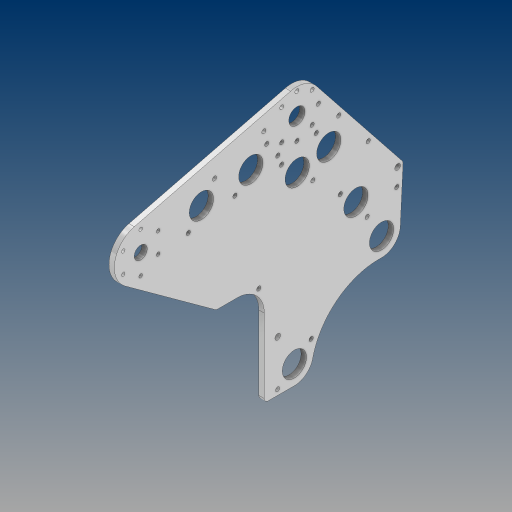
# Autodesk Inventor part: Intake Roller Plate
Saved by Autodesk Inventor 2024.3 (Build 283343000, 343)
## iProperties
Created: 2024-07-25
Part Number: Intake Roller Plate
Material: Aluminum 6061
Document SubType Name: Modeling
Designer: Kenji
Density: 2.7 g/cm^3
Appearance: Aluminum - Dark
Author: Kenji
Autodesk Inventor part; units mm, degrees
ref_plane "YZ Plane" through (0, 0, 0) normal (1, 0, 0) x (0, 1, 0)
ref_plane "XZ Plane" through (0, 0, 0) normal (0, 1, 0) x (-1, 0, 0)
ref_plane "XY Plane" through (0, 0, 0) normal (0, 0, 1) x (1, 0, 0)
sketch "Sketch1" plane through (0, 0, 0) normal (1, 0, 0) x (0, 1, 0)
  line L0 (127, 0) -> (127, -31.75) construction
  line L1 (95.25, -63.5) -> (31.75, -63.5) construction
  line L2 (0, -31.75) -> (0, 0) construction
  arc A0 (95.25, -63.5) -> (127, -31.75) centre (95.25, -31.75) ccw construction
  arc A1 (0, -31.75) -> (31.75, -63.5) centre (31.75, -31.75) ccw construction
  line L3 (0, 0) -> (0, 19.05) construction
  line L4 (0, 19.05) -> (-12.7, 19.05) construction
  line L5 (82.55, 19.05) -> (82.55, 292.1) construction
  circle A2 centre (82.55, 292.1) radius 25.4 construction
  circle A3 centre (82.55, 292.1) radius 31.75 construction
  circle A4 centre (231.775, 292.1) radius 25.4 construction
  circle A5 centre (231.775, 292.1) radius 31.75 construction
  line L6 (-12.7, 19.05) -> (82.55, 19.05) construction
  line L7 (127, 0) -> (0, 0) construction
  line L8 (-12.7, 19.05) -> (-12.7, -285.75) construction
  circle A6 centre (38.1, -172.5837) radius 50.8 construction
  circle A7 centre (104.9083, -202.0677) radius 25.4 construction
  circle A8 centre (104.9083, -202.0677) radius 14.2875
  circle A9 centre (154.8209, -171.8196) radius 25.4 construction
  circle A10 centre (154.8209, -171.8196) radius 14.2875
  circle A11 centre (250.0002, -47.5843) radius 22.225 construction
  circle A12 centre (250.0002, -47.5843) radius 25.4 construction
  circle A13 centre (250.0002, -47.5843) radius 14.2875
  line L9 (82.55, 19.05) -> (127, 19.05) construction
  line L10 (127, 19.05) -> (127, 0) construction
  circle A14 centre (154.8209, -171.8196) radius 22.225 construction
  circle A15 centre (104.9083, -202.0677) radius 22.225 construction
  circle A16 centre (25.4, -99.06) radius 25.4 construction
  circle A17 centre (25.4, -99.06) radius 23.8125 construction
  line L11 (25.4, -73.66) -> (25.4, -63.5) construction
  circle A18 centre (219.8086, -102.3786) radius 25.4 construction
  circle A19 centre (219.8086, -102.3786) radius 22.225 construction
  circle A20 centre (219.8086, -102.3786) radius 14.2875
  line L12 (0, -99.06) -> (-12.7, -99.06) construction
  circle A21 centre (63.172, -79.375) radius 6.477 construction
  circle A22 centre (25.4, -99.06) radius 14.2875
  circle A23 centre (63.172, -79.375) radius 3.2512
  circle A24 centre (95.1707, -129.6948) radius 50.8 construction
  circle A25 centre (147.0613, -96.0158) radius 50.8 construction
  circle A26 centre (105.4747, -117.9903) radius 50.8 construction
  circle A27 centre (166.1747, -221.0415) radius 3.2512
  circle A28 centre (242.3971, 10.8357) radius 14.2875
  circle A29 centre (242.3971, 10.8357) radius 22.225 construction
  line L13 (219.8086, -102.3786) -> (154.8209, -171.8196) construction
  line L14 (154.8209, -171.8196) -> (104.9083, -202.0677) construction
  line L15 (82.55, 19.05) -> (31.75, 19.05) construction
  line L16 (31.75, 19.05) -> (31.75, 292.1) construction
  line L17 (31.75, 292.1) -> (82.55, 292.1) construction
  circle A30 centre (242.3971, 10.8357) radius 7.62 construction
  line L18 (-12.7, -285.75) -> (571.5, -285.75) construction
  line L19 (571.5, -285.75) -> (571.5, 292.1) construction
  line L20 (31.75, 292.1) -> (571.5, 292.1) construction
  line L21 (127, 19.05) -> (571.5, 19.05) construction
  circle A31 centre (230.3321, 82.55) radius 7.62
  circle A32 centre (230.3321, 82.55) radius 23.8125 construction
  circle A33 centre (254.1446, 82.55) radius 2.0828
  circle A34 centre (230.3321, 82.55) radius 27.94 construction
  circle A35 centre (230.3321, 82.55) radius 31.115 construction
  circle A36 centre (242.2384, 103.1722) radius 2.0828
  circle A37 centre (218.4259, 103.1722) radius 2.0828
  circle A38 centre (206.5196, 82.55) radius 2.0828
  circle A39 centre (218.4259, 61.9278) radius 2.0828
  circle A40 centre (242.2384, 61.9278) radius 2.0828
  line L22 (-12.7, -63.5) -> (368.3, -63.5) construction
  circle A41 centre (166.1747, -221.0415) radius 6.4262 construction
  line L23 (368.3, -63.5) -> (368.3, -285.75) construction
  circle A42 centre (63.172, -79.375) radius 6.35 construction
  circle A43 centre (242.3971, 10.8357) radius 25.4 construction
  line L24 (242.3971, 10.8357) -> (250.0002, -47.5843) construction
  line L25 (82.55, 19.05) -> (141.3002, 19.05) construction
  line L26 (141.3002, 19.05) -> (141.3002, 209.55) construction
  line L27 (141.3002, 209.55) -> (82.55, 209.55) construction
  line L28 (82.55, 209.55) -> (82.55, 19.05) construction
  circle A44 centre (133.35, 12.7) radius 6.35 construction
  circle A45 centre (177.4795, -39.017) radius 50.8 construction
  circle A46 centre (177.8, -23.221) radius 50.8 construction
  circle A47 centre (25.4, -99.06) radius 22.225 construction
  line L29 (3.175, -99.06) -> (3.175, -68.2752)
  circle A48 centre (133.35, 12.7) radius 3.2512 construction
  arc A49 (166.1747, -227.4677) -> (170.1786, -226.0679) centre (166.1747, -221.0415) ccw
  arc A50 (3.175, -99.06) -> (20.3984, -120.7149) centre (25.4, -99.06) ccw
  arc A51 (7.9502, -63.5) -> (3.175, -68.2752) centre (7.9502, -68.2752) ccw
  arc A52 (260.5134, 90.1152) -> (205.1617, 100.8419) centre (230.3321, 82.55) ccw
  line L30 (141.3002, 53.086) -> (157.9626, 53.086) construction
  line L31 (157.9626, 53.086) -> (157.9626, 86.106) construction
  line L32 (157.9626, 86.106) -> (141.3002, 86.106) construction
  line L33 (141.3002, 86.106) -> (141.3002, 53.086) construction
  line L34 (232.868, -28.832) -> (267.1324, -66.3365) construction
  circle A53 centre (232.868, -28.832) radius 2.4257
  circle A54 centre (267.1324, -66.3365) radius 2.4257
  line L35 (236.3587, 15.4834) -> (262.5254, -4.6567) construction
  line L36 (236.3587, 15.4834) -> (222.2689, 26.3281) construction
  circle A55 centre (262.5254, -4.6567) radius 2.4257
  circle A56 centre (222.2689, 26.3281) radius 2.4257
  circle A57 centre (262.5254, -4.6567) radius 6.35 construction
  circle A58 centre (222.2689, 26.3281) radius 6.35 construction
  circle A59 centre (232.868, -28.832) radius 6.35 construction
  circle A60 centre (267.1324, -66.3365) radius 6.35 construction
  line L37 (219.8086, -102.3786) -> (237.1646, -83.8332) construction
  line L38 (219.8086, -102.3786) -> (202.4526, -120.9239) construction
  circle A61 centre (237.1646, -83.8332) radius 2.4257
  circle A62 centre (202.4526, -120.9239) radius 2.4257
  circle A63 centre (172.1769, -153.2743) radius 2.4257
  circle A64 centre (133.0985, -184.9838) radius 2.4257
  arc A65 (82.6927, -201.4208) -> (103.7686, -224.2634) centre (104.9083, -202.0677) ccw
  circle A66 centre (9.525, -79.2321) radius 2.4257
  circle A67 centre (9.525, -79.2321) radius 6.35 construction
  arc A68 (82.6927, -201.4208) -> (20.3984, -120.7149) centre (2.2987, -199.0799) ccw
  line L39 (9.525, -79.2321) -> (41.275, -118.8879) construction
  circle A69 centre (41.275, -118.8879) radius 2.4257
  circle A70 centre (41.275, -118.8879) radius 5.6007 construction
  line L40 (7.9502, -63.5) -> (95.25, -63.5)
  arc A71 (95.25, -63.5) -> (127, -31.75) centre (95.25, -31.75) ccw
  line L41 (166.1747, -227.4677) -> (103.7686, -224.2634)
  line L42 (104.9083, -202.0677) -> (83.1859, -215.2319) construction
  line L43 (82.55, 133.35) -> (88.9, 133.35) construction
  line L44 (82.55, 184.15) -> (88.9, 184.15) construction
  line L45 (127, -31.75) -> (127, -8.2637)
  line L46 (127.9123, -5.4564) -> (205.1617, 100.8419)
  arc A72 (127.9123, -5.4564) -> (127, -8.2637) centre (131.7752, -8.2637) ccw
  line L47 (82.55, 44.45) -> (571.5, 44.45) construction
  circle A73 centre (133.0985, -184.9838) radius 6.35 construction
  circle A74 centre (141.7169, -99.98) radius 50.8 construction
  circle A75 centre (277.7476, -102.0288) radius 30 construction
  circle A76 centre (277.7476, -102.0288) radius 25.4 construction
  circle A77 centre (303.1476, -102.0288) radius 2.3876
  circle A78 centre (295.7081, -84.0683) radius 2.3876
  circle A79 centre (277.7476, -76.6288) radius 2.3876 construction
  circle A80 centre (259.7871, -84.0683) radius 2.3876
  circle A81 centre (252.3476, -102.0288) radius 2.3876
  circle A82 centre (259.7871, -119.9893) radius 2.3876
  circle A83 centre (277.7476, -127.4288) radius 2.3876
  circle A84 centre (295.7081, -119.9893) radius 2.3876
  circle A85 centre (277.7476, -102.0288) radius 9.525
  circle A86 centre (219.8086, -102.3786) radius 19.05 construction
  circle A87 centre (227.4601, -139.7023) radius 19.05 construction
  circle A88 centre (227.4601, -139.7023) radius 14.2875
  line L48 (247.7482, -102.2099) -> (245.2082, -102.2252) construction
  line L49 (170.1786, -226.0679) -> (296.4391, -125.4942)
  line L50 (260.5134, 90.1152) -> (306.8474, -94.7347)
  arc A89 (296.4391, -125.4942) -> (306.8474, -94.7347) centre (277.7476, -102.0288) ccw
  circle A90 centre (219.8086, -102.3786) radius 30.48 construction
  circle A91 centre (277.7476, -102.0288) radius 30.48 construction
  circle A92 centre (248.6408, -79.4624) radius 3.81 construction
  line L51 (251.6519, -81.7968) -> (253.6592, -83.3531) construction
  line L52 (245.6582, -81.833) -> (243.6698, -83.4134) construction
  circle A93 centre (248.6408, -79.4624) radius 2.3812
  circle A94 centre (248.9154, -124.945) radius 3.81 construction
  circle A95 centre (248.9154, -124.945) radius 2.3876
  line L53 (251.898, -122.5744) -> (253.8865, -120.9939) construction
  line L54 (245.9043, -122.6105) -> (243.897, -121.0542) construction
  line L55 (248.6408, -75.6524) -> (248.6408, -72.9479) construction
  line L56 (219.8086, -102.3786) -> (219.8086, -88.0911) construction
  circle A96 centre (232.868, -28.832) radius 2.4257
  circle A97 centre (9.525, -79.2321) radius 2.4257
  circle A98 centre (146.08, -220.0775) radius 2.4257
  circle A99 centre (253.6387, -151.4689) radius 2.4257
  circle A100 centre (209.9304, -186.285) radius 2.4257
  circle A101 centre (281.6771, -62.9926) radius 2.4257
  line L57 (123.7263, -57.0623) -> (232.868, -28.832) construction
  line L58 (232.868, -28.832) -> (281.6771, -62.9926) construction
  line L59 (281.6771, -62.9926) -> (253.6387, -151.4689) construction
  line L60 (253.6387, -151.4689) -> (209.9304, -186.285) construction
  line L61 (209.9304, -186.285) -> (146.08, -220.0775) construction
  line L62 (146.08, -220.0775) -> (9.525, -79.2321) construction
  line L63 (123.7263, -57.0623) -> (9.525, -79.2321) construction
  circle A102 centre (146.08, -220.0775) radius 6.35 construction
  circle A103 centre (123.7263, -57.0623) radius 2.4257
  line L64 (277.7476, -102.0288) -> (219.8086, -102.3786) construction
  line L65 (250.0002, -47.5843) -> (219.8086, -102.3786) construction
  point P0 (-12.7, -172.5837)
  point P1 (180.2209, -171.8196)
  point P2 (104.775, 19.05)
  point P3 (172.6009, -221.0415)
  point P4 (127, -63.5)
  point P5 (3.175, -63.5)
  point P6 (104.9083, -227.4677)
  point P7 (95.25, -63.5)
  point P8 (127, -6.7118)
  point P9 (222.7121, 82.55)
  point P10 (220.1721, 10.8357)
  point P11 (25.4, -99.06)
  dimension "d58" = 101.6
  dimension "d267" = 15.24
  dimension "d283" = 15.24
  dimension "d284" = 47.625
  dimension "d523" = 50.8
  dimension "d2" = 31.75
  dimension "d3" = 19.05
  dimension "d4" = 12.7
  dimension "d7" = 273.05
  dimension "d8" = 50.8
  dimension "d9" = 6.35
  dimension "d10" = 50.8
  dimension "d11" = 6.35
  dimension "d12" = 149.225
  dimension "d14" = 127
  dimension "d16" = 304.8
  dimension "d175" = 31.75
  dimension "d180" = 50.8
  dimension "d181" = 1.5875
  dimension "d187" = 31.75
  dimension "d189" = 12.7
  dimension "d191" = 12.954
  dimension "d192" = 28.575
  dimension "d201" = 6.5024
  dimension "d207" = 101.6
  dimension "d208" = 101.6
  dimension "d210" = 130.175
  dimension "d214" = 15.875
  dimension "d218" = 6.5024
  dimension "d220" = 143.1895
  dimension "d236" = 50.8
  dimension "d237" = 44.45
  dimension "d271" = 584.2
  dimension "d285" = 4.1656
  dimension "d290" = 55.88
  dimension "d292" = 3.175
  dimension "d321" = 360
  dimension "d323" = 381
  dimension "d328" = 3.175
  dimension "d336" = 12.7
  dimension "d375" = 10.16
  dimension "d388" = 50.8
  dimension "d389" = 3.175
  dimension "d395" = 44.45
  dimension "d399" = 58.7502
  dimension "d400" = 190.5
  dimension "d404" = 12.7
  dimension "d405" = 101.6
  dimension "d406" = 101.6
  dimension "d407" = 58.42
  dimension "d409" = 3.175
  dimension "d410" = 6.5024
  dimension "d411" = 4.7752
  dimension "d427" = 16.6624
  dimension "d428" = 33.02
  dimension "d429" = 34.036
  dimension "d433" = 4.8514
  dimension "d434" = 4.8514
  dimension "d435" = 4.8514
  dimension "d436" = 4.8514
  dimension "d441" = 45
  dimension "d443" = 4.8514
  dimension "d444" = 4.8514
  dimension "d445" = 4.8514
  dimension "d446" = 4.8514
  dimension "d453" = 4.8514
  dimension "d459" = 4.8514
  dimension "d460" = 3.175
  dimension "d470" = 273.05
  constraints: 133 end point, 97 centre point, 60 point on circle, 38 tangent, 36 point on line, 29 coincident, 16 equal radius, 16 perpendicular, 14 horizontal alignment, 12 concentric, 6 collinear, 6 horizontal, 6 parallel, 6 vertical, 5 midpoint, 4 equal length, 3 vertical alignment, 53 other
  measures "d2" radius of A0
  measures "d3" distance of L2.end L3.end
  measures "d4" distance of L3.end L4.end
  measures "d7" distance of L5.start L5.end
  measures "d8" diameter of A2
  measures "d9" radial gap between concentric circles of A2 A3
  measures "d10" diameter of A4
  measures "d11" radial gap between concentric circles of A4 A5
  measures "d12" distance of L17.end A4.centre
  measures "d14" distance of L0.start L2.end
  measures "d16" distance of L4.end L8.end
  measures "d175" radius of A1
  measures "d180" diameter of A16
  measures "d181" radial gap between concentric circles of A16 A17
  measures "d187" distance of L0.start L0.end
  measures "d189" distance of L12.start L12.end
  measures "d191" diameter of A21
  measures "d192" diameter of A22
  measures "d201" diameter of A23
  measures "d207" diameter of A24
  measures "d208" diameter of A25
  measures "d210" distance of A21.centre A14.centre
  measures "d214" distance from line of L1 A21.centre
  measures "d218" diameter of A27
  measures "d220" distance of A0.centre A19.centre
  measures "d236" distance of L5.start L15.end
  measures "d237" distance of L4.end L15.end
  measures "d271" distance of L8.end L18.end
  measures "d285" diameter of A33
  measures "d290" diameter of A34
  measures "d292" radial gap between concentric circles of A34 A35
  measures "d323" distance of L22.start L22.end
  measures "d328" radial gap between concentric circles of A27 A41
  measures "d336" diameter of A42
  measures "d375" distance of L11.start L11.end
  measures "d388" diameter of A9
  measures "d389" radial gap between concentric circles of A15 A7
  measures "d395" diameter of A15
  measures "d399" distance of L27.end L26.end
  measures "d400" distance of L26.end L25.end
  measures "d404" diameter of A44
  measures "d405" diameter of A45
  measures "d406" diameter of A46
  measures "d407" vertical distance of L24.start L24.end
  measures "d409" radial gap between concentric circles of A16 A47
  measures "d410" diameter of A48
  measures "d411" radius of A51
  measures "d427" distance of L32.end L31.end
  measures "d428" distance between parallel lines of L30 L32
  measures "d429" distance from line of L25.end L30
  measures "d433" diameter of A53
  measures "d434" diameter of A54
  measures "d435" diameter of A55
  measures "d436" diameter of A56
  measures "d441" angle of L24 L35
  measures "d443" diameter of A61
  measures "d444" diameter of A62
  measures "d445" diameter of A63
  measures "d446" diameter of A64
  measures "d453" diameter of A66
  measures "d459" diameter of A69
  measures "d460" radial gap between concentric circles of A69 A70
  measures "d470" distance of L19.end L21.end
extrude "Extrusion14" add sketch "Sketch1" along normal blind 6.35 contours L29 A51 L40 A71 L45 A72 L46 A52 L50 A89 L49 A49 L41 A65 A68 A50 | A77 | A81 | A83 | A93 | A95 | A98 | A99 | A100 | A101 | A103
extrude "Extrusion15" cut sketch "Sketch1" along normal blind 6.35 contours A77 | A81 | A83
extrude "Extrusion16" cut sketch "Sketch1" along normal blind 6.35 contours A93 | A95
extrude "Extrusion17" cut sketch "Sketch1" along normal blind 25.4 contours A98 | A99 | A100 | A101 | A103
body "Solid13"
